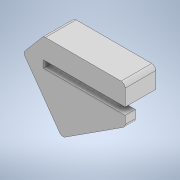
# Autodesk Inventor part: tapeStopper
Saved by Autodesk Inventor 2022.3 (Build 263350030, 350C)
## iProperties
Created: 2022-11-22
Part Number: tapeStopper
Material: Generic
Document SubType Name: Modeling
Designer: yiunf
Density: 1 g/cm^3
Appearance: Default
Author: yiunf
## iProperties of the stored document tapeStopper_3DPrint.ipt
Created: 2022-11-22
Part Number: tapeStopper_3DPrint
Material: Generic
Document SubType Name: Modeling
Designer: yiunf
Density: 1 g/cm^3
Appearance: Default
Author: yiunf
Autodesk Inventor part; units mm, degrees
ref_plane "YZ Plane" through (0, 0, 0) normal (1, 0, 0) x (0, 1, 0)
ref_plane "XZ Plane" through (0, 0, 0) normal (0, 1, 0) x (-1, 0, 0)
ref_plane "XY Plane" through (0, 0, 0) normal (0, 0, 1) x (1, 0, 0)
sketch "Sketch1" plane through (0, 0, 0) normal (0, 0, 1) x (1, 0, 0)
  line L0 (0, 0) -> (4, 0)
  line L1 (4, 0) -> (4, -5)
  line L2 (4, -5) -> (0, -5)
  line L3 (0, -5) -> (0, 0)
  line L4 (0, -5) -> (-5, -5)
  line L5 (-5, -5) -> (-5, 0)
  line L6 (-5, 0) -> (0, 0)
  line L7 (0, 0) -> (0, -5)
  line L8 (-5, 0) -> (0, 0)
  line L9 (0, 0) -> (0, 3.5)
  line L10 (0, 3.5) -> (-5, 3.5)
  line L11 (-5, 3.5) -> (-5, 0)
  line L12 (-5, 3.5) -> (35, 3.5)
  line L13 (35, 3.5) -> (35, 13.5)
  line L14 (35, 13.5) -> (-5, 13.5)
  line L15 (-5, 13.5) -> (-5, 3.5)
  line L16 (-5, 1.75) -> (-15, 1.75)
  line L17 (-15, 1.75) -> (-5, 13.5)
  line L18 (-15, 1.75) -> (-5, -5)
  dimension "d0" = 4
  dimension "d1" = 5
  dimension "d2" = 5
  dimension "d3" = 3.5
  dimension "d4" = 40
  dimension "d5" = 10
  dimension "d6" = 10
  constraints: 38 end point, 8 parallel, 5 horizontal, 4 perpendicular, 1 midpoint
  measures "d0" distance of L1.end L2.end
  measures "d1" distance of L0.end L1.end
  measures "d2" distance of L5.end L6.end
  measures "d3" distance of L9.end L8.end
  measures "d4" distance of L14.end L13.end
  measures "d5" distance of L13.end L12.end
  measures "d6" distance of L16.start L16.end
extrude "Extrusion1" add sketch "Sketch1" along normal blind 15 contours L0 L1 L2 L3 | L3 L4 L5 L6 | L5 L18 L16 L11 | L10 L15 L14 L13 L12 | L16 L17 L15 L11
sketch "Sketch2" plane through (0, 0, 15) normal (0, 0, 1) x (1, 0, 0)
  line L0 (4, -5) -> (4, 0) projected
  line L1 (4, 0) -> (35, 0)
  line L2 (35, 0) -> (35, -5)
  line L3 (35, -5) -> (4, -5)
  line L4 (4, -5) -> (4, 0)
  line L5 (4, -5) -> (4, -25)
  line L6 (-15, 1.75) -> (-5, -5) projected
  line L7 (4, -25) -> (-15, 1.75)
  line L8 (-5, -5) -> (4, -5) projected
  line L9 (-15, 1.75) -> (-5, -5)
  line L10 (-5, -5) -> (4, -5)
  line L11 (4, -25) -> (35, -5)
  point P0 (0, 0)
  dimension "d9" = 5
  dimension "d13" = 20
  constraints: 18 end point, 2 parallel, 1 horizontal, 1 perpendicular, 1 vertical
  measures "d9" distance of L1.end L2.end
  measures "d13" distance of L3.end L5.end
extrude "Extrusion2" add sketch "Sketch2" against normal blind 5
fillet "Fillet1" radius 2 8 edges at (-15, 1.75, 5) (-15, 1.75, 12.5) (-5, 13.5, 7.5) (4, -5, 5) (35, -5, 12.5) (-5, -5, 5) (35, 13.5, 7.5) (4, -25, 12.5)
body "Solid1"
